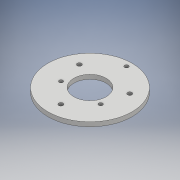
# Autodesk Inventor part: SUPORT STEEP
Saved by Autodesk Inventor 2018 (Build 220112000, 112)
## iProperties
Created: 2018-03-05
Part Number: SUPORT STEEP
Material: Generic
Document SubType Name: Modeling
Designer: isai
Density: 1 g/cm^3
Appearance: Default
Author: isai
Autodesk Inventor part; units mm, degrees
ref_plane "YZ Plane" through (0, 0, 0) normal (1, 0, 0) x (0, 1, 0)
ref_plane "XZ Plane" through (0, 0, 0) normal (0, 1, 0) x (-1, 0, 0)
ref_plane "XY Plane" through (0, 0, 0) normal (0, 0, 1) x (1, 0, 0)
sketch "Sketch1" plane through (0, 0, 0) normal (0, 0, 1) x (1, 0, 0)
  circle A0 centre (0, 0) radius 39
  circle A1 centre (0, -27) radius 2
  circle A2 centre (23.3827, 13.5) radius 2
  circle A3 centre (-23.3827, 13.5) radius 2
  circle A4 centre (0, 0) radius 15
  dimension "d2" = 4
  dimension "d3" = 27
  dimension "d4" = 360
  dimension "d5" = 30
  dimension "d12" = 78
  constraints: 5 centre point, 1 coincident, 7 other
  measures "d2" diameter of A1
  measures "d3" distance of point (0, 0) A1.centre
  measures "d5" diameter of A4
  measures "d12" diameter of A0
extrude "Extrusion1" add sketch "Sketch1" along normal blind 4
sketch "Sketch4" plane through (0, 0, 4) normal (0, 0, 1) x (1, 0, 0)
  circle A0 centre (0, 33.9) radius 1.8
  circle A1 centre (-18.3848, -8.4848) radius 1.8
  circle A2 centre (18.3848, -8.4848) radius 1.8
  circle A3 centre (0, 0) radius 39
  circle A4 centre (-23.3827, 13.5) radius 1.5001
  circle A5 centre (0, -27) radius 1.5001
  circle A6 centre (23.3827, 13.5) radius 1.5001
  constraints: 7 centre point
extrude "Extrusion4" cut sketch "Sketch4" against normal blind 4 contours A0 | A1 | A2
body "Solid1"
